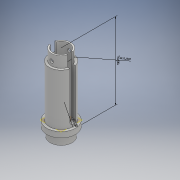
# Autodesk Inventor part: canon
Saved by Autodesk Inventor 2018 (Build 220112000, 112)
## iProperties
Created: 2018-02-07
Part Number: canon
Material: Générique
Document SubType Name: Modeling
Designer: Mephiro
Density: 1 g/cm^3
Appearance: Par défaut
Author: Mephiro
Autodesk Inventor part; units mm, degrees
ref_plane "YZ Plane" through (0, 0, 0) normal (1, 0, 0) x (0, 1, 0)
ref_plane "XZ Plane" through (0, 0, 0) normal (0, 1, 0) x (-1, 0, 0)
ref_plane "XY Plane" through (0, 0, 0) normal (0, 0, 1) x (1, 0, 0)
sketch "Esquisse1" plane through (0, 0, 0) normal (0, 0, 1) x (1, 0, 0)
  circle A0 centre (0, 0) radius 8.75
  circle A1 centre (0, 0) radius 7.5
  dimension "d0" = 17.5
  dimension "d1" = 15
  constraints: 2 centre point, 2 coincident
  measures "d0" diameter of A0
  measures "d1" diameter of A1
extrude "Extrusion1" add sketch "Esquisse1" against normal blind 10
sketch "Esquisse2" plane through (0, 0, -10) normal (0, 0, -1) x (-1, 0, 0)
  circle A0 centre (0, 0) radius 10.75
  dimension "d4" = 21.5
  constraints: 1 centre point, 1 coincident
  measures "d4" diameter of A0
extrude "Extrusion2" add sketch "Esquisse2" along normal blind 60
sketch "Esquisse3" plane through (0, 0, -70) normal (0, 0, -1) x (-1, 0, 0)
  circle A0 centre (0, 0) radius 7.5
  dimension "d7" = 15
  constraints: 1 centre point, 1 coincident
  measures "d7" diameter of A0
extrude "Extrusion3" cut sketch "Esquisse3" against normal blind 60
ref_plane "Plan de construction1" through (0, 0, -57) normal (0, 0, 1) x (1, 0, 0)
sketch "Esquisse4" plane through (0, 0, -57) normal (0, 0, 1) x (1, 0, 0)
  circle A0 centre (0, 0) radius 13
  circle A1 centre (0, 0) radius 10
  dimension "d12" = 26
  dimension "d13" = 20
  constraints: 2 centre point, 2 coincident
  measures "d12" diameter of A0
  measures "d13" diameter of A1
extrude "Extrusion4" add sketch "Esquisse4" against normal blind 5
sketch "Esquisse5" plane through (0, 0, 0) normal (0, 0, 1) x (1, 0, 0)
  line L0 (-15.0714, 2.5) -> (16.7857, 2.5)
  line L1 (16.7857, 2.5) -> (16.7857, -2.5)
  line L2 (16.7857, -2.5) -> (-15.0714, -2.5)
  line L3 (-15.0714, -2.5) -> (-15.0714, 2.5)
  point P0 (0, 0)
  dimension "d16" = 5
  dimension "d17" = 2.5
  constraints: 8 end point, 2 parallel, 1 horizontal, 1 perpendicular
  measures "d16" distance of L0.end L1.end
  measures "d17" distance from line of L2 point (0, 0)
extrude "Extrusion5" cut sketch "Esquisse5" against normal blind 55
fillet "Congé1" radius 2.5 4 edges at (8.7632, 2.5, -55) (-8.7632, 2.5, -55) (8.7632, -2.5, -55) (-8.7632, -2.5, -55)
sketch "Esquisse6" plane through (0, 0, 0) normal (0, 1, 0) x (-1, 0, 0)
  circle A0 centre (0, -6) radius 1.6
  line L0 (-8.3853, 0) -> (8.3853, 0) projected
  point P0 (0, 0)
  dimension "d21" = 3.2
  dimension "d22" = 6
  constraints: 1 centre point
  measures "d21" diameter of A0
  measures "d22" distance from line of L0 A0.centre
extrude "Extrusion6" cut sketch "Esquisse6" along normal mid plane 20
sketch "Esquisse8" plane through (0, 0, -70) normal (0, 0, -1) x (-1, 0, 0)
  circle A0 centre (0, 0) radius 11.0733
  circle A1 centre (0, 0) radius 10
  dimension "d36" = 20
  constraints: 2 centre point, 2 coincident
  measures "d36" diameter of A1
extrude "Extrusion7" cut sketch "Esquisse8" against normal blind 10
